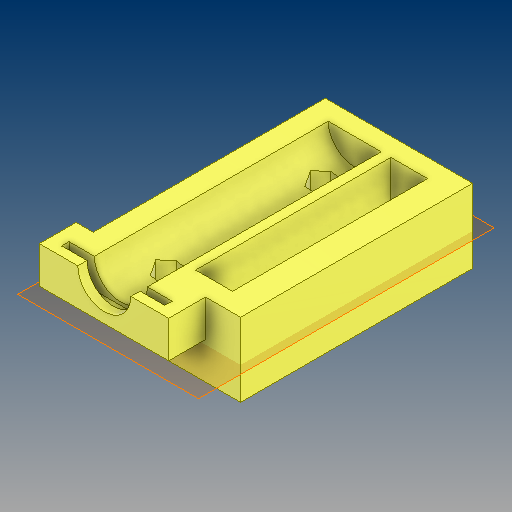
# Autodesk Inventor part: uchwyt_strzykawka_srodek_proba_zapisania
Saved by Autodesk Inventor 2021 (Build 250183000, 183)
## iProperties
Created: 2022-05-16
Part Number: uchwyt_strzykawka_srodek_proba_zapisania
Material: PC/ABS Plastic
Document SubType Name: Modeling
Designer: agnpi
Density: 0.357273 g/cm^3
Appearance: Smooth - Yellow
Author: agnpi
Autodesk Inventor part; units mm, degrees
ref_plane "YZ Plane" through (0, 0, 0) normal (1, 0, 0) x (0, 1, 0)
ref_plane "XZ Plane" through (0, 0, 0) normal (0, 1, 0) x (-1, 0, 0)
ref_plane "XY Plane" through (0, 0, 0) normal (0, 0, 1) x (1, 0, 0)
sketch "Sketch1" plane through (0, 0, 0) normal (0, 1, 0) x (-1, 0, 0)
  line L0 (28, 0) -> (-28, 0) projected
  line L1 (0, -44.1) -> (0, 44.1) projected
  line L2 (-20, 31.5) -> (20, 31.5)
  line L3 (20, 31.5) -> (20, -31.5)
  line L4 (20, -31.5) -> (-20, -31.5)
  line L5 (-20, -31.5) -> (-20, 31.5)
  line L6 (-20, 31.5) -> (20, -31.5) construction
  line L7 (20, 31.5) -> (-20, -31.5) construction
  point P0 (0, 0)
  dimension "d0" = 40
  dimension "d1" = 63
  constraints: 12 end point, 2 midpoint, 2 parallel, 1 horizontal, 1 perpendicular
  measures "d0" distance of L3.end L4.end
  measures "d1" distance of L2.end L3.end
extrude "Extrusion1" add sketch "Sketch1" along normal blind 20
sketch "Sketch2" plane through (0, 20, 0) normal (0, 1, 0) x (1, 0, 0)
  line L0 (20, 31.5) -> (-20, 31.5) projected
  line L1 (-20, 31.5) -> (-20, -31.5) projected
  line L2 (2.8, 26.5) -> (12.8, 26.5)
  line L3 (12.8, 26.5) -> (12.8, -26.5)
  line L4 (12.8, -26.5) -> (2.8, -26.5)
  line L5 (2.8, -26.5) -> (2.8, 26.5)
  line L6 (20, -31.5) -> (20, 31.5) projected
  dimension "d9" = 10
  dimension "d10" = 53
  dimension "d11" = 5
  dimension "d23" = 7.2
  constraints: 8 end point, 2 parallel, 1 horizontal, 1 perpendicular
  measures "d9" distance of L3.end L4.end
  measures "d10" distance of L2.end L3.end
  measures "d11" distance between parallel lines of L0 L2
  measures "d23" distance between parallel lines of L6 L3
extrude "Extrusion2" cut sketch "Sketch2" against normal blind 11
sketch "Sketch3" plane through (0, 9, 0) normal (0, 1, 0) x (1, 0, 0)
  line L0 (20, -31.5) -> (20, 31.5) projected
  line L1 (12.8, 26.5) -> (12.8, -26.5) projected
  line L2 (20, 31.5) -> (-20, 31.5) projected
  point P0 (0, 0)
  point P1 (7.8, 14.41)
  point P2 (7.8, -14.3)
  dimension "d22" = 5
  dimension "d27" = 17.09
  dimension "d40" = 28.71
  dimension "d41" = 12.2
  measures "d22" distance from line of L1 point (7.8, 14.41)
  measures "d27" distance from line of L2 point (7.8, 14.41)
  measures "d40" distance of point (7.8, 14.41) point (7.8, -14.3)
  measures "d41" distance from line of L0 point (7.8, -14.3)
hole "Hole1" at (7.8, 9, -14.41) at (7.8, 9, 14.3) direction (0, -1, 0) diameter 3.242 end through all thread size "M4x0.7" class "6H" standard "ISO Metric profile"
sketch "Sketch5" plane through (0, 9, 0) normal (0, 1, 0) x (1, 0, 0)
  circle A0 centre (7.8, 14.41) radius 1.621 projected
  line L0 (9.8207, 10.91) -> (5.7793, 10.91)
  line L1 (5.7793, 10.91) -> (3.7585, 14.41)
  line L2 (3.7585, 14.41) -> (5.7793, 17.91)
  line L3 (5.7793, 17.91) -> (9.8207, 17.91)
  line L4 (9.8207, 17.91) -> (11.8415, 14.41)
  line L5 (11.8415, 14.41) -> (9.8207, 10.91)
  line L6 (2.8, 26.5) -> (12.8, 26.5) projected
  line L7 (12.8, -26.5) -> (2.8, -26.5) projected
  circle A1 centre (7.8, -14.3) radius 1.621 projected
  line L8 (9.8207, -17.8) -> (5.7793, -17.8)
  line L9 (5.7793, -17.8) -> (3.7585, -14.3)
  line L10 (3.7585, -14.3) -> (5.7793, -10.8)
  line L11 (5.7793, -10.8) -> (9.8207, -10.8)
  line L12 (9.8207, -10.8) -> (11.8415, -14.3)
  line L13 (11.8415, -14.3) -> (9.8207, -17.8)
  point P0 (0, 0)
  dimension "d37" = 7
  dimension "d42" = 7
  constraints: 24 end point, 4 parallel, 2 coincident, 26 other
  measures "d37" distance between parallel lines of L0 L3
  measures "d42" distance between parallel lines of L8 L11
extrude "Extrusion3" cut sketch "Sketch5" against normal blind 4 contours L0 L1 L2 L3 L4 L5 | A1 | L8 L9 L10 L11 L12 L13
sketch "Sketch9" plane through (-20, 0, 31.5) normal (0, 0, 1) x (1, 0, 0)
  line L0 (30.47, 20) -> (30.47, 10)
  line L1 (30.47, 10) -> (-4.63, 10)
  line L2 (-4.63, 10) -> (-4.63, 20)
  line L3 (0, 0) -> (0, 20) projected
  line L4 (40, 20) -> (0, 20) projected
  arc A0 (5.8, 20) -> (20.2, 20) centre (13, 20) ccw
  line L5 (-4.63, 20) -> (5.8, 20)
  line L6 (20.2, 20) -> (30.47, 20)
  line L7 (40, 0) -> (40, 20) projected
  line L8 (5.8, 20) -> (20.2, 20)
  point P0 (20, 0)
  point P1 (0, 10)
  dimension "d58" = 35.1
  dimension "d59" = 10
  dimension "d60" = 4.63
  dimension "d64" = 7.2
  dimension "d65" = 17.63
  dimension "d66" = 19.8
  dimension "d67" = 14.4
  constraints: 12 end point, 3 parallel, 2 horizontal, 2 perpendicular, 2 point on circle, 1 centre point, 1 point on line
  measures "d58" distance of L0.end L1.end
  measures "d59" distance of L0.start L0.end
  measures "d60" distance between parallel lines of L3 L2
  measures "d64" radius of A0
  measures "d65" distance from line of L2 A0.centre
  measures "d66" distance from line of L7 L6.start
  measures "d67" distance of L6.start L5.end
extrude "Extrusion6" add sketch "Sketch9" along normal blind 10 contours L0 L1 L3 L4 A0 | L1 L2 L5 L3
extrude "Extrusion7" cut sketch "Sketch9" against normal blind 58 contours A0 L4
sketch "Sketch10" plane through (0, 20, 0) normal (0, 1, 0) x (1, 0, 0)
  line L0 (-21.08, -37) -> (6.92, -37)
  line L1 (6.92, -37) -> (6.92, -39)
  line L2 (6.92, -39) -> (-21.08, -39)
  line L3 (-21.08, -39) -> (-21.08, -37)
  line L4 (0.2, -41.5) -> (-14.2, -41.5) projected
  line L5 (-24.63, -31.5) -> (-24.63, -41.5) projected
  point P0 (0, 0)
  dimension "d72" = 2
  dimension "d73" = 2.5
  dimension "d74" = 28
  dimension "d75" = 3.55
  constraints: 8 end point, 2 parallel, 1 horizontal, 1 perpendicular
  measures "d72" distance between parallel lines of L2 L0
  measures "d73" distance between parallel lines of L4 L2
  measures "d74" distance of L1.end L2.end
  measures "d75" distance from line of L5 L0.start
extrude "Extrusion8" cut sketch "Sketch10" against normal blind 8
sketch "Sketch13" plane through (0, 0, 0) normal (0, -1, 0) x (1, 0, 0)
  line L0 (-20, -31.5) -> (-20, 31.5) projected
  line L1 (20, -31.5) -> (-20, -31.5) projected
  point P0 (0, 0)
  point P1 (-7, -18.5)
  dimension "d89" = 13
  dimension "d90" = 13
  measures "d89" distance from line of L0 point (-7, -18.5)
  measures "d90" distance from line of L1 point (-7, -18.5)
ref_plane "Work Plane3" through (0, 8.8, 0) normal (0, 1, 0) x (1, 0, 0)
sketch "Sketch31" plane through (0, 8.8, 0) normal (0, 1, 0) x (1, 0, 0)
  line L0 (-4.9793, 15) -> (-9.0207, 15)
  line L1 (-9.0207, 15) -> (-11.0415, 18.5)
  line L2 (-11.0415, 18.5) -> (-9.0207, 22)
  line L3 (-9.0207, 22) -> (-4.9793, 22)
  line L4 (-4.9793, 22) -> (-2.9585, 18.5)
  line L5 (-2.9585, 18.5) -> (-4.9793, 15)
  line L6 (20, 31.5) -> (-20, 31.5) projected
  line L7 (-20, 31.5) -> (-20, -31.5) projected
  line L8 (-4.9793, -27) -> (-9.0207, -27)
  line L9 (-9.0207, -27) -> (-11.0415, -23.5)
  line L10 (-11.0415, -23.5) -> (-9.0207, -20)
  line L11 (-9.0207, -20) -> (-4.9793, -20)
  line L12 (-4.9793, -20) -> (-2.9585, -23.5)
  line L13 (-2.9585, -23.5) -> (-4.9793, -27)
  point P0 (0, 0)
  point P1 (-7, 18.5)
  point P2 (-7, -23.5)
  dimension "d159" = 13
  dimension "d160" = 13
  dimension "d161" = 7
  dimension "d171" = 7
  dimension "d172" = 13
  dimension "d173" = 42
  constraints: 24 end point, 3 parallel, 26 other
  measures "d159" distance from line of L6 point (-7, 18.5)
  measures "d160" distance from line of L7 point (-7, 18.5)
  measures "d161" distance between parallel lines of L0 L3
  measures "d171" distance between parallel lines of L8 L11
  measures "d172" distance from line of L7 point (-7, -23.5)
  measures "d173" distance of point (-7, 18.5) point (-7, -23.5)
extrude "Extrusion19" cut sketch "Sketch31" along normal through all
hole "Hole7" at (-7, 0, -18.5) direction (0, 1, 0) diameter 3.242 end through all thread size "M4x0.7" class "6H" standard "ISO Metric profile"
sketch "Sketch33" plane through (0, 8.8, 0) normal (0, 1, 0) x (1, 0, 0)
  line L0 (-20, 31.5) -> (-20, -31.5) projected
  line L1 (-9.0207, -20) -> (-4.9793, -20) projected
  point P0 (0, 0)
  point P1 (-7, -23.5001)
  dimension "d181" = 13
  dimension "d182" = 3.5001
  measures "d181" distance from line of L0 point (-7, -23.5)
  measures "d182" distance from line of L1 point (-7, -23.5)
hole "Hole8" at (-7, 8.8, 23.5001) direction (0, -1, 0) diameter 3.242 end through all thread size "M4x0.7" class "6H" standard "ISO Metric profile"
body "Solid1"
